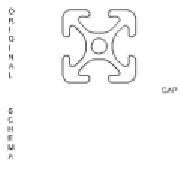
# Autodesk Inventor part: CAP 0_0_370_03_000   Profil 5  20x20 natur
Saved by Autodesk Inventor 2016 (Build 200138000, 138)
## iProperties
IsCustomPart: 1
Company: CAP
Created: 2015-12-11
Part Number: CAP 0_0_370_03_000   Profil 5  20x20 natur
Material: Al Mg Si 0,5 F 25     3.3206.72  warmausgehärtet (natur)
Description: CAP 0_0_370_03_000   Profil 5  20x20 natur  S1
Document SubType Name: Modeling
Designer: 4ndreas
Manufacturer: CAP
Standards Organization: CAP
Language: de-DE
Size Designation: CAP 0_0_370_03_000   Profil 5  20x20 natur
Categories: <MemberInstance><Categories><Category DisplayName="Profile" InternalName="089c4875-fa83-4c05-b084-43b9cc11f5ed" Mnemonic="GRDR"><CategoryParameter DisplayName="Masse pro Längeneinheit" InternalName="0bb95a10-148f-4027-a459-38d7b056702a" Mnemonic="shpmass"/><CategoryParameter DisplayName="Querschnittsfläche" InternalName="1ff91680-64b0-4202-b9a3-7fd3f94bba3b" Mnemonic="secarea"/><CategoryParameter DisplayName="Trägheitsradius (x)" InternalName="25778675-03e9-40c1-b6a8-4a9ed693320d" Mnemonic="gyrradx"/><CategoryParameter DisplayName="Torsion-Festigkeitsmodul" InternalName="26c1ec35-5026-4c63-ad0a-751cf684a536" Mnemonic="torrigmod"/><CategoryParameter DisplayName="Abstand zum Schwerpunkt X-X" InternalName="26c9bdb8-9c79-4b4f-a92e-8e197583c9c4" Mnemonic="grcendistX"/><CategoryParameter DisplayName="Alte Varianten-ID" InternalName="340afe4f-75d7-48d3-ab7d-943f3c3da468" Mnemonic="LegacyMemberID"/><CategoryParameter DisplayName="Basislänge" InternalName="42e34263-8f20-4d0e-ad48-bf1385b87c24" Mnemonic="shplen"/><CategoryParameter DisplayName="Trägheitsmoment (y)" InternalName="4b9f58ea-bced-460e-81ea-3d29ca5a49e3" Mnemonic="inermomy"/><CategoryParameter DisplayName="Trägheitsmoment (x)" InternalName="4cd780bc-73d7-43ac-917a-579e5cbd684d" Mnemonic="inermomx"/><CategoryParameter DisplayName="Benutzerdefinierter Basispunkt" InternalName="4f1d1b73-316d-484b-a3df-9cbabb16eb77" Mnemonic="shpBasePoint"/><CategoryParameter DisplayName="Objekthöhe" InternalName="50274e7d-5ac0-4796-92cb-c59e54983c67" Mnemonic="shpheig"/><CategoryParameter DisplayName="Widerstandsmoment (y)" InternalName="59eaa5e9-d227-48dc-b6c1-6920f96e0f95" Mnemonic="secmody"/><CategoryParameter DisplayName="Schnittbezeichnung" InternalName="5a64d034-428d-49c8-ba32-7619764de20f" Mnemonic="shpdes"/><CategoryParameter DisplayName="Widerstandsmoment (x)" InternalName="72cfad18-cf51-4ed4-aaa7-c6b224f8419f" Mnemonic="secmodx"/><CategoryParameter DisplayName="Drehrissmodul" InternalName="7c55a8dc-8844-49f9-a867-cc677b30ec9a" Mnemonic="torsecmod"/><CategoryParameter DisplayName="Objektbreite" InternalName="7c717d54-a18f-4666-b4d4-573cce22c62c" Mnemonic="shpwdth"/><CategoryParameter DisplayName="Zweite Objektdicke" InternalName="9251a8e1-85fd-4e47-af99-afdb762317d9" Mnemonic="shpthick2"/><CategoryParameter DisplayName="GG Erstellt" InternalName="9c666724-f362-4ea7-ac62-f6a007de5c69" Mnemonic="shpFGAuto"/><CategoryParameter DisplayName="Abstand zum Schwerpunkt Y-Y" InternalName="bcc4fb17-7af4-436a-8f8c-d0aa3b0248c5" Mnemonic="grcendistY"/><CategoryParameter DisplayName="Trägheitsradius (y)" InternalName="bfa18ebe-1636-4dbe-8d42-b263e0b73184" Mnemonic="gyrrady"/><CategoryParameter DisplayName="Objektdicke" InternalName="d109cf76-8eb4-42fc-9800-4409734adc67" Mnemonic="shpthick"/><CategoryParameter DisplayName="Koeffizient für Schubverschiebung" InternalName="de4c90c6-aaa8-468f-a335-6737b311b5d3" Mnemonic="shdispc"/><Category DisplayName="CAP" InternalName="b2b813c8-4dc8-4eec-8dba-86b6d4c2b5a1" Mnemonic="CAP"/></Category><Category DisplayName="Datentyp" InternalName="23b78d0f-2648-40c6-8793-ca6db495c9e8" Mnemonic="DATATYPE"><CategoryParameter DisplayName="Anzeigename" InternalName="05415f3d-3907-474b-a020-eb9d644f4cf3" Mnemonic="DISPLAYNAME"/><CategoryParameter DisplayName="Norm" InternalName="0c0a119c-1e12-4c84-803f-101930972f5e" Mnemonic="STANDARD"/><CategoryParameter DisplayName="Beschreibung" InternalName="13903e3d-64b1-4950-80da-f627842ea37f" Mnemonic="DESCRIPTION"/><CategoryParameter DisplayName="Bezeichnung" InternalName="2675968c-4ce5-49e0-a4f5-552d29089031" Mnemonic="DESIGNATION"/><CategoryParameter DisplayName="Standardzeile" InternalName="2af9ec52-faaa-4026-b378-f9fa4afca842" Mnemonic="DEFAULTROW"/><CategoryParameter DisplayName="Ordnername" InternalName="3f06958e-8713-4116-9be7-ed6184ecc97b" Mnemonic="FOLDERNAME"/><CategoryParameter DisplayName="Revisionsanleitung" InternalName="45a75005-10b1-4dfc-8d6d-dfe629f0b93c" Mnemonic="REVISIONGUID"/><CategoryParameter DisplayName="Dateiname" InternalName="8b46a4cc-9585-4fed-90c3-899f57e09a73" Mnemonic="FILENAME"/><CategoryParameter DisplayName="Normungsorganisation" InternalName="8f5914e1-4693-403f-8ab5-d37768198c9d" Mnemonic="STDSORG"/><CategoryParameter DisplayName="Gruppenversion" InternalName="914462f6-6e19-4b14-ba84-155b9680b1d0" Mnemonic="FAMILYREVISION"/><CategoryParameter DisplayName="Normrevision" InternalName="91d5a463-65c2-4fde-b823-3b7fea5e8e17" Mnemonic="STANDARDREVISION"/><CategoryParameter DisplayName="Variantenrevision" InternalName="a65d44b9-392f-4f4f-857b-e4b3d54996fe" Mnemonic="MEMBERREVISION"/><CategoryParameter DisplayName="ClipFormat" InternalName="bc51e27b-3422-4e78-93ef-cec197ddf230" Mnemonic="CLIPFORMAT"/><CategoryParameter DisplayName="Hersteller" InternalName="cd6c7a72-a28a-4e50-99a9-2c7f4e13e5ad" Mnemonic="MANUFACTURER"/><CategoryParameter DisplayName="InternerName" InternalName="cf1d0246-76d9-4b4a-8305-fa0409afb5c1" Mnemonic="INTERNALNAME"/><CategoryParameter DisplayName="IstMetrisch" InternalName="e2385c5b-1ea4-4823-96a8-8de651266ec3" Mnemonic="ISMETRIC"/><Category DisplayName="Bauteil" InternalName="c0e0b642-3bcb-4cc8-9e80-f96d35c4afa4" Mnemonic="PART"><CategoryParameter DisplayName="Bauteilnummer" InternalName="016b6077-bfbe-49bd-92c9-d8d59c39c941" Mnemonic="PARTNUMBER"/><CategoryParameter DisplayName="Bestandsnummer" InternalName="4dba7c1c-e26c-444e-836c-b08b433409a8" Mnemonic="STOCKNUMBER"/><CategoryParameter DisplayName="Materialschlüssel" InternalName="5c9a8adb-dd2b-4535-b97f-0a94a95fe41f" Mnemonic="MATERIALKEY"/><CategoryParameter DisplayName="Material" InternalName="818a152a-d3c3-49ca-80ee-df7d91421b8e" Mnemonic="MATERIAL"/></Category></Category></Categories><FamilyTemplate Id="CAP 0_0_370_03_000   Profil 5  20x20 natur"><FamilyTemplateParameters><FamilyTemplateParameter ObjectType="kModelParameterObject" ValueType="xs:double" Id="12" ObjectReferenceKey="L0"/><FamilyTemplateParameter ObjectType="kPartComponentDefinitionObject" ValueType="xs:string" Id="23" SubObjectId="Material"/><FamilyTemplateParameter ObjectType="kPropertyObject" ValueType="xs:string" Id="26" ObjectReferenceKey="{32853F0F-3444-11d1-9E93-0060B03C1CA6}" SubObjectId="5"/><FamilyTemplateParameter ObjectType="kPropertyObject" ValueType="xs:string" Id="27" ObjectReferenceKey="{32853F0F-3444-11d1-9E93-0060B03C1CA6}" SubObjectId="52"/></FamilyTemplateParameters></FamilyTemplate><CategoryParameterMap><ParamToTemplateMap><ParamToTemplate CategoryParameter="//CategoryParameter[@InternalName='cf1d0246-76d9-4b4a-8305-fa0409afb5c1']" ConstantValue="bf077d1e-0d56-4bf4-9b9d-c13fcf92694b"/><ParamToTemplate CategoryParameter="//CategoryParameter[@InternalName='45a75005-10b1-4dfc-8d6d-dfe629f0b93c']" ConstantValue="e01d2531-348a-4692-bcdb-523ff43b41e7"/><ParamToTemplate CategoryParameter="//CategoryParameter[@InternalName='3f06958e-8713-4116-9be7-ed6184ecc97b']" ConstantValue="CAP 0_0_370_03_000   Profil 5  20x20 natur  S1"/><ParamToTemplate CategoryParameter="//CategoryParameter[@InternalName='8f5914e1-4693-403f-8ab5-d37768198c9d']" ConstantValue="CAP"/><ParamToTemplate CategoryParameter="//CategoryParameter[@InternalName='0c0a119c-1e12-4c84-803f-101930972f5e']" TemplateParameter="18"/><ParamToTemplate CategoryParameter="//CategoryParameter[@InternalName='91d5a463-65c2-4fde-b823-3b7fea5e8e17']" TemplateParameter="19"/><ParamToTemplate CategoryParameter="//CategoryParameter[@InternalName='cd6c7a72-a28a-4e50-99a9-2c7f4e13e5ad']" ConstantValue="CAP"/><ParamToTemplate CategoryParameter="//CategoryParameter[@InternalName='13903e3d-64b1-4950-80da-f627842ea37f']" ConstantValue="CAP 0_0_370_03_000   Profil 5  20x20 natur  S1"/><ParamToTemplate CategoryParameter="//CategoryParameter[@InternalName='05415f3d-3907-474b-a020-eb9d644f4cf3']" ConstantValue="Profil 5  20x20 natur  S1"/><ParamToTemplate CategoryParameter="//CategoryParameter[@InternalName='914462f6-6e19-4b14-ba84-155b9680b1d0']" ConstantValue="11"/><ParamToTemplate CategoryParameter="//CategoryParameter[@InternalName='bc51e27b-3422-4e78-93ef-cec197ddf230']" ConstantValue="CF_INVENTOR.STDPARTS"/><ParamToTemplate CategoryParameter="//CategoryParameter[@InternalName='e2385c5b-1ea4-4823-96a8-8de651266ec3']" ConstantValue="true"/><ParamToTemplate CategoryParameter="//CategoryParameter[@InternalName='2af9ec52-faaa-4026-b378-f9fa4afca842']" ConstantValue="1"/><ParamToTemplate CategoryParameter="//CategoryParameter[@InternalName='9c666724-f362-4ea7-ac62-f6a007de5c69']" ConstantValue="1"/><ParamToTemplate CategoryParameter="//CategoryParameter[@InternalName='8b46a4cc-9585-4fed-90c3-899f57e09a73']" ConstantValue="CAP 0_0_370_03_000   Profil 5  20x20 natur-"/><ParamToTemplate CategoryParameter="//CategoryParameter[@InternalName='a65d44b9-392f-4f4f-857b-e4b3d54996fe']" ConstantValue="f741cc97-694d-41ec-a21e-c6308bc0fed2"/><ParamToTemplate CategoryParameter="//CategoryParameter[@InternalName='a65d44b9-392f-4f4f-857b-e4b3d54996fe']" ConstantValue="f741cc97-694d-41ec-a21e-c6308bc0fed2"/><ParamToTemplate CategoryParameter="//CategoryParameter[@InternalName='2675968c-4ce5-49e0-a4f5-552d29089031']" TemplateParameter="27"/><ParamToTemplate CategoryParameter="//CategoryParameter[@InternalName='42e34263-8f20-4d0e-ad48-bf1385b87c24']" TemplateParameter="12"/><ParamToTemplate CategoryParameter="//CategoryParameter[@InternalName='818a152a-d3c3-49ca-80ee-df7d91421b8e']" TemplateParameter="23"/><ParamToTemplate CategoryParameter="//CategoryParameter[@InternalName='016b6077-bfbe-49bd-92c9-d8d59c39c941']" TemplateParameter="26"/></ParamToTemplateMap></CategoryParameterMap></MemberInstance>
Stock Number: CAP 0_0_370_03_000   Profil 5  20x20 natur
Mass: 42.1645 g
Surface Area: 146.813 cm^2
Volume: 15.6272 cm^3
Density: 2.69815 g/cm^3
Appearance: Aluminium - dunkel
G_L: 85,000 mm
Author: 4ndreas
Autodesk Inventor part; units mm, degrees
ref_plane "YZ Plane" through (0, 0, 0) normal (1, 0, 0) x (0, 1, 0)
ref_plane "Endebene" through (0, 0, 85) normal (0, 0, 1) x (1, 0, 0)
ref_plane "Startebene" through (0, 0, 0) normal (0, 0, 1) x (1, 0, 0)
sketch "Skizze1" plane through (0, 0, 0) normal (0, 0, 1) x (1, 0, 0)
  line L0 (2.8753, 8.4384) -> (2.877, 8.434)
  line L1 (2.8747, 8.4384) -> (2.8753, 8.4384)
  line L2 (2.877, 8.434) -> (2.877, 8.4368)
  line L3 (2.873, 8.434) -> (2.8747, 8.4384)
  line L4 (2.877, 8.4368) -> (2.8776, 8.4368)
  line L5 (2.8715, 8.434) -> (2.873, 8.434)
  line L6 (2.8776, 8.4368) -> (2.8776, 8.436)
  arc A0 (2.8706, 8.4349) -> (2.8715, 8.434) centre (2.8715, 8.4349) ccw
  line L7 (2.8776, 8.436) -> (2.8785, 8.436)
  line L8 (2.8706, 8.4369) -> (2.8706, 8.4349)
  arc A1 (2.8785, 8.436) -> (2.8785, 8.4378) centre (2.8785, 8.4369) ccw
  arc A2 (2.8715, 8.4378) -> (2.8706, 8.4369) centre (2.8715, 8.4369) ccw
  line L9 (2.8785, 8.4378) -> (2.8776, 8.4378)
  line L10 (2.873, 8.4378) -> (2.8715, 8.4378)
  line L11 (2.8776, 8.4378) -> (2.8776, 8.4369)
  line L12 (2.873, 8.4384) -> (2.873, 8.4378)
  line L13 (2.8776, 8.4369) -> (2.877, 8.4369)
  line L14 (2.8715, 8.4384) -> (2.873, 8.4384)
  line L15 (2.877, 8.4369) -> (2.877, 8.4384)
  arc A3 (2.8715, 8.4384) -> (2.87, 8.4369) centre (2.8715, 8.4369) ccw
  line L16 (2.877, 8.4384) -> (2.8785, 8.4384)
  line L17 (2.87, 8.4349) -> (2.87, 8.4369)
  arc A4 (2.8785, 8.4354) -> (2.8785, 8.4384) centre (2.8785, 8.4369) ccw
  arc A5 (2.87, 8.4349) -> (2.8715, 8.4334) centre (2.8715, 8.4349) ccw
  line L18 (2.8785, 8.4354) -> (2.8776, 8.4354)
  line L19 (2.8734, 8.4334) -> (2.8715, 8.4334)
  line L20 (2.8776, 8.4354) -> (2.8776, 8.4334)
  line L21 (2.8742, 8.4354) -> (2.8734, 8.4334)
  line L22 (2.8776, 8.4334) -> (2.8766, 8.4334)
  line L23 (2.875, 8.4354) -> (2.8742, 8.4354)
  line L24 (2.8766, 8.4334) -> (2.8758, 8.4354)
  line L25 (2.875, 8.436) -> (2.875, 8.4354)
  line L26 (2.8758, 8.4354) -> (2.8751, 8.4354)
  line L27 (2.8744, 8.436) -> (2.875, 8.436)
  line L28 (2.8751, 8.4354) -> (2.8751, 8.436)
  line L29 (2.875, 8.4375) -> (2.8744, 8.436)
  line L30 (2.8751, 8.436) -> (2.8756, 8.436)
  line L31 (2.8756, 8.436) -> (2.875, 8.4375)
  arc A6 (-9.4142, 9.4142) -> (-10, 8) centre (-8, 8) ccw
  line L32 (-10, 8) -> (-10, 3.375)
  arc A7 (-10, 3.375) -> (-9.2, 2.575) centre (-9.2, 3.375) ccw
  line L33 (-9.2, 2.575) -> (-8.4359, 2.575)
  arc A8 (-8.4359, 2.575) -> (-8.1359, 2.8788) centre (-8.4359, 2.875) ccw
  line L34 (-8.1359, 2.8788) -> (-8.1618, 4.9477)
  arc A9 (-6.7962, 5.5234) -> (-8.1618, 4.9477) centre (-7.3619, 4.9577) ccw
  line L35 (-6.7962, 5.5234) -> (-4.5287, 3.2559)
  arc A10 (-3.65, 1.1346) -> (-4.5287, 3.2559) centre (-6.65, 1.1346) ccw
  line L36 (-3.65, 1.1346) -> (-3.65, 0)
  line L37 (-3.65, 0) -> (-3.65, -1.1346)
  arc A11 (-4.5287, -3.2559) -> (-3.65, -1.1346) centre (-6.65, -1.1346) ccw
  line L38 (-4.5287, -3.2559) -> (-6.7962, -5.5234)
  arc A12 (-8.1618, -4.9477) -> (-6.7962, -5.5234) centre (-7.3619, -4.9577) ccw
  line L39 (-8.1618, -4.9477) -> (-8.1359, -2.8788)
  arc A13 (-8.1359, -2.8788) -> (-8.4359, -2.575) centre (-8.4359, -2.875) ccw
  line L40 (-8.4359, -2.575) -> (-9.2, -2.575)
  arc A14 (-9.2, -2.575) -> (-10, -3.375) centre (-9.2, -3.375) ccw
  line L41 (-10, -3.375) -> (-10, -8)
  arc A15 (-10, -8) -> (-9.4142, -9.4142) centre (-8, -8) ccw
  arc A16 (-9.4142, -9.4142) -> (-8, -10) centre (-8, -8) ccw
  line L42 (-8, -10) -> (-3.375, -10)
  arc A17 (-3.375, -10) -> (-2.575, -9.2) centre (-3.375, -9.2) ccw
  line L43 (-2.575, -9.2) -> (-2.575, -8.4359)
  arc A18 (-2.575, -8.4359) -> (-2.8788, -8.1359) centre (-2.875, -8.4359) ccw
  line L44 (-2.8788, -8.1359) -> (-4.9477, -8.1618)
  arc A19 (-5.5234, -6.7962) -> (-4.9477, -8.1618) centre (-4.9577, -7.3619) ccw
  line L45 (-5.5234, -6.7962) -> (-3.2559, -4.5287)
  arc A20 (-1.1346, -3.65) -> (-3.2559, -4.5287) centre (-1.1346, -6.65) ccw
  line L46 (-1.1346, -3.65) -> (0, -3.65)
  line L47 (0, -3.65) -> (1.1346, -3.65)
  arc A21 (3.2559, -4.5287) -> (1.1346, -3.65) centre (1.1346, -6.65) ccw
  line L48 (3.2559, -4.5287) -> (5.5234, -6.7962)
  arc A22 (4.9477, -8.1618) -> (5.5234, -6.7962) centre (4.9577, -7.3619) ccw
  line L49 (4.9477, -8.1618) -> (2.8788, -8.1359)
  arc A23 (2.8788, -8.1359) -> (2.575, -8.4359) centre (2.875, -8.4359) ccw
  line L50 (2.575, -8.4359) -> (2.575, -9.2)
  arc A24 (2.575, -9.2) -> (3.375, -10) centre (3.375, -9.2) ccw
  line L51 (3.375, -10) -> (8, -10)
  arc A25 (8, -10) -> (9.4142, -9.4142) centre (8, -8) ccw
  arc A26 (9.4142, -9.4142) -> (10, -8) centre (8, -8) ccw
  line L52 (10, -8) -> (10, -3.375)
  arc A27 (10, -3.375) -> (9.2, -2.575) centre (9.2, -3.375) ccw
  line L53 (9.2, -2.575) -> (8.4359, -2.575)
  arc A28 (8.4359, -2.575) -> (8.1359, -2.8788) centre (8.4359, -2.875) ccw
  line L54 (8.1359, -2.8788) -> (8.1618, -4.9477)
  arc A29 (6.7962, -5.5234) -> (8.1618, -4.9477) centre (7.3619, -4.9577) ccw
  line L55 (6.7962, -5.5234) -> (4.5287, -3.2559)
  arc A30 (3.65, -1.1346) -> (4.5287, -3.2559) centre (6.65, -1.1346) ccw
  line L56 (3.65, -1.1346) -> (3.65, 0)
  line L57 (3.65, 0) -> (3.65, 1.1346)
  arc A31 (4.5287, 3.2559) -> (3.65, 1.1346) centre (6.65, 1.1346) ccw
  line L58 (4.5287, 3.2559) -> (6.7962, 5.5234)
  arc A32 (8.1618, 4.9477) -> (6.7962, 5.5234) centre (7.3619, 4.9577) ccw
  line L59 (8.1618, 4.9477) -> (8.1359, 2.8788)
  arc A33 (8.1359, 2.8788) -> (8.4359, 2.575) centre (8.4359, 2.875) ccw
  line L60 (8.4359, 2.575) -> (9.2, 2.575)
  arc A34 (9.2, 2.575) -> (10, 3.375) centre (9.2, 3.375) ccw
  line L61 (10, 3.375) -> (10, 8)
  arc A35 (10, 8) -> (9.4142, 9.4142) centre (8, 8) ccw
  arc A36 (9.4142, 9.4142) -> (8, 10) centre (8, 8) ccw
  line L62 (8, 10) -> (3.375, 10)
  arc A37 (3.375, 10) -> (2.575, 9.2) centre (3.375, 9.2) ccw
  line L63 (2.575, 9.2) -> (2.575, 8.4359)
  arc A38 (2.575, 8.4359) -> (2.8788, 8.1359) centre (2.875, 8.4359) ccw
  line L64 (2.8788, 8.1359) -> (4.9477, 8.1618)
  arc A39 (5.5234, 6.7962) -> (4.9477, 8.1618) centre (4.9577, 7.3619) ccw
  line L65 (5.5234, 6.7962) -> (3.2559, 4.5287)
  arc A40 (1.1346, 3.65) -> (3.2559, 4.5287) centre (1.1346, 6.65) ccw
  line L66 (1.1346, 3.65) -> (0, 3.65)
  line L67 (0, 3.65) -> (-1.1346, 3.65)
  arc A41 (-3.2559, 4.5287) -> (-1.1346, 3.65) centre (-1.1346, 6.65) ccw
  line L68 (-3.2559, 4.5287) -> (-5.5234, 6.7962)
  arc A42 (-4.9477, 8.1618) -> (-5.5234, 6.7962) centre (-4.9577, 7.3619) ccw
  line L69 (-4.9477, 8.1618) -> (-2.8788, 8.1359)
  arc A43 (-2.8788, 8.1359) -> (-2.575, 8.4359) centre (-2.875, 8.4359) ccw
  line L70 (-2.575, 8.4359) -> (-2.575, 9.2)
  arc A44 (-2.575, 9.2) -> (-3.375, 10) centre (-3.375, 9.2) ccw
  line L71 (-3.375, 10) -> (-8, 10)
  arc A45 (-8, 10) -> (-9.4142, 9.4142) centre (-8, 8) ccw
  arc A46 (-2.15, 0) -> (-1.5203, -1.5203) centre (0, 0) ccw
  arc A47 (-1.5203, -1.5203) -> (0, -2.15) centre (0, 0) ccw
  arc A48 (0, -2.15) -> (1.5203, -1.5203) centre (0, 0) ccw
  arc A49 (1.5203, -1.5203) -> (2.15, 0) centre (0, 0) ccw
  arc A50 (2.15, 0) -> (1.5203, 1.5203) centre (0, 0) ccw
  arc A51 (1.5203, 1.5203) -> (0, 2.15) centre (0, 0) ccw
  arc A52 (0, 2.15) -> (-1.5203, 1.5203) centre (0, 0) ccw
  arc A53 (-1.5203, 1.5203) -> (-2.15, 0) centre (0, 0) ccw
  constraints: 144 end point, 108 point on circle, 54 centre point, 27 horizontal, 22 vertical, 258 other
extrude "Körper" add sketch "Skizze1" along normal up to surface (85 mm away) from surface at 0 contours A45 L71 A44 L70 A43 L69 A42 L68 A41 L67 L66 A40 L65 A39 L64 A38 L63 A37 L62 A36 A35 L61 A34 L60 A33 L59 A32 L58 A31 L57 L56 A30 L55 A29 L54 A28 L53 A27 L52 A26 A25 L51 A24 L50 A23 L49 A22 L48 A21 L47 L46 A20 L45 A19 L44 A18 L43 A17 L42 A16 A15 L41 A14 L40 A13 L39 A12 L38 A11 L37 L36 A10 L35 A9 L34 A8 L33 A7 L32 A6
sketch "Skizze2" plane through (0, 0, 0) normal (0, 0, 1) x (1, 0, 0)
  line L0 (0, 0) -> (10, 0)
ref_plane "Arbeitsebene3" through (0, 0, 0) normal (0, -1, 0) x (1, 0, 0)
sketch "Skizze3" plane through (0, 0, 0) normal (0, -1, 0) x (1, 0, 0)
  line L0 (-2, 0) -> (12, 0)
  line L1 (-2, 85) -> (12, 85)
  dimension "d7" = 85
  measures "d7" distance between parallel lines of L0 L1
equation "\"G_OFFSET_START\" = 0"
equation "\"G_OFFSET_END\" = 0"
equation "\"d3\" = L0 + G_OFFSET_END"
equation "\"G_L\" = d7"
equation "\"L0\" = 85"
